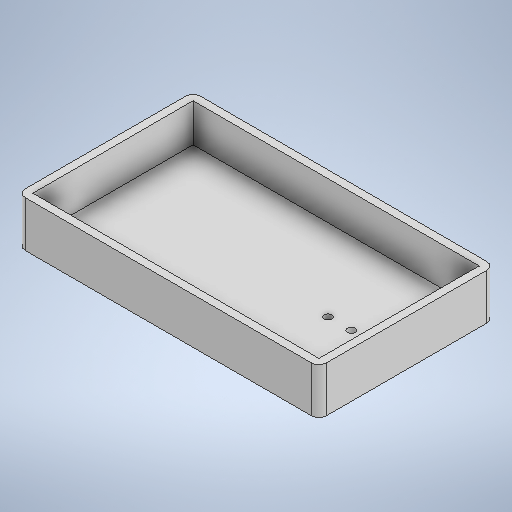
# Autodesk Inventor part: SimpleElectronicBox
Saved by Autodesk Inventor 2025.2 (Build 292293000, 293)
## iProperties
Created: 2026-02-18
Part Number: SimpleElectronicBox
Material: Generic
Document SubType Name: Modeling
Designer: sanku
Density: 1 g/cm^3
Appearance: Default
Author: sanku
Autodesk Inventor part; units mm, degrees
ref_plane "YZ Plane" through (0, 0, 0) normal (1, 0, 0) x (0, 1, 0)
ref_plane "XZ Plane" through (0, 0, 0) normal (0, 1, 0) x (-1, 0, 0)
ref_plane "XY Plane" through (0, 0, 0) normal (0, 0, 1) x (1, 0, 0)
sketch "Sketch1" plane through (0, 0, 0) normal (0, 1, 0) x (-1, 0, 0)
  line L0 (0, 0) -> (-238.125, 0)
  line L1 (-238.125, 0) -> (-238.125, -133.35)
  line L2 (-238.125, -133.35) -> (0, -133.35)
  line L3 (0, -133.35) -> (0, 0)
  line L4 (0, 6.35) -> (-237.998, 6.35)
  line L5 (-244.475, -0.127) -> (-244.475, -133.35)
  line L6 (-238.125, -139.7) -> (-0.1245, -139.7)
  line L7 (6.35, -133.35) -> (6.35, 0)
  arc A0 (-0.1245, -139.7) -> (6.35, -133.35) centre (-0.1245, -133.2243) ccw
  arc A1 (6.35, 0) -> (-0.1245, 6.35) centre (-0.1258, -0.127) ccw
  arc A2 (-244.475, -133.2243) -> (-238.125, -139.7) centre (-237.998, -133.2242) ccw
  arc A3 (-237.998, 6.35) -> (-244.475, -0.127) centre (-237.998, -0.127) ccw
  dimension "d0" = 238.125
  dimension "d1" = 133.35
  dimension "d2" = 6.35
  dimension "d9" = 6.477
  dimension "d10" = 6.477
  dimension "d11" = 6.477
  constraints: 16 end point, 8 point on circle, 5 point on line, 4 centre point, 4 parallel, 2 perpendicular, 1 horizontal, 1 tangent
  measures "d0" distance of L2.end L1.end
  measures "d1" distance of L1.end L0.end
  measures "d2" distance between parallel lines of L3 L7
  measures "d9" radius of A1
  measures "d10" radius of A2
  measures "d11" radius of A3
extrude "Extrusion1" add sketch "Sketch1" along normal blind 38.1
sketch "Sketch2" plane through (0, 0, 0) normal (0, -1, 0) x (1, 0, 0)
  line L0 (0, 0) -> (238.125, 0)
  line L1 (238.125, 0) -> (238.125, -133.35)
  line L2 (238.125, -133.35) -> (0, -133.35)
  line L3 (0, -133.35) -> (0, 0)
  dimension "d5" = 238.125
  dimension "d6" = 133.35
  constraints: 8 end point, 2 parallel, 1 horizontal, 1 perpendicular
  measures "d5" distance of L1.end L2.end
  measures "d6" distance of L0.end L1.end
extrude "Extrusion2" add sketch "Sketch2" against normal blind 6.35
sketch "Sketch7" plane through (0, 6.35, 0) normal (0, 1, 0) x (1, 0, 0)
  line L0 (237.998, 0) -> (155.448, 0)
  line L1 (238.125, 0) -> (0, 0) projected
  line L2 (155.448, 0) -> (155.448, 57.15)
  line L3 (155.448, 57.15) -> (237.998, 57.15)
  circle A0 centre (218.3382, 65.3946) radius 3.175
  circle A1 centre (199.6313, 65.4249) radius 3.175
  line L4 (218.3382, 65.3946) -> (180.2382, 65.3946)
  circle A2 centre (180.2382, 65.3946) radius 3.175
  dimension "d31" = 82.55
  dimension "d32" = 57.15
  dimension "d33" = 6.35
  dimension "d36" = 6.35
  dimension "d37" = 38.1
  dimension "d38" = 6.35
  constraints: 8 end point, 3 centre point, 2 perpendicular, 1 horizontal, 1 point on line
  measures "d31" distance of L0.start L0.end
  measures "d32" distance of L0.end L2.end
  measures "d33" diameter of A0
  measures "d36" diameter of A1
  measures "d37" distance of L4.start L4.end
  measures "d38" diameter of A2
extrude "Extrusion4" cut sketch "Sketch7" against normal blind 6.35
equation "\"d34\" = d38"
body "Solid1"
